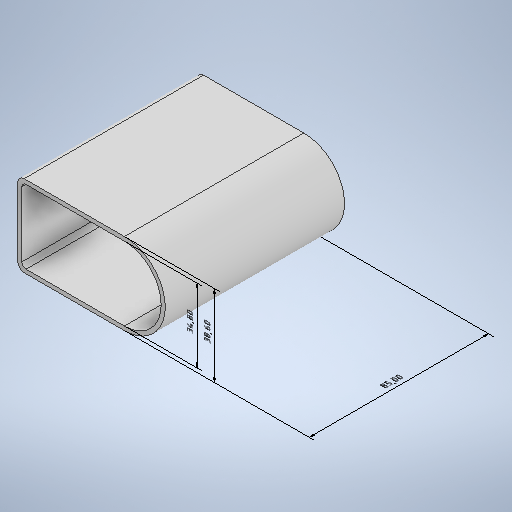
# Autodesk Inventor part: víko
Saved by Autodesk Inventor 2025.3 (Build 293356000, 356)
## iProperties
Created: 2025-06-12
Part Number: víko
Material: Generic
Document SubType Name: Modeling
Designer: Repete
Density: 1 g/cm^3
Appearance: Default
Author: Repete
Autodesk Inventor part; units mm, degrees
ref_plane "YZ Plane" through (0, 0, 0) normal (1, 0, 0) x (0, 1, 0)
ref_plane "XZ Plane" through (0, 0, 0) normal (0, 1, 0) x (-1, 0, 0)
ref_plane "XY Plane" through (0, 0, 0) normal (0, 0, 1) x (1, 0, 0)
sketch "Sketch1" plane through (0, 0, 0) normal (0, 1, 0) x (-1, 0, 0)
  line L0 (35.4, 17.4) -> (35.4, -17.4)
  line L1 (35.4, -17.4) -> (-13.2013, -17.4)
  arc A0 (-13.2013, 17.4) -> (-13.2013, -17.4) centre (-13.2013, 0) ccw
  line L2 (-13.2013, 17.4) -> (35.4, 17.4)
  line L3 (37.3, -19.3) -> (37.3, 19.3)
  line L4 (37.3, 19.3) -> (-13.2013, 19.3)
  arc A1 (-13.2013, 19.3) -> (-13.2013, -19.3) centre (-13.2013, 0) ccw
  line L5 (-13.2013, -19.3) -> (37.3, -19.3)
  point P0 (0, 0)
  point P1 (-13.2013, 0)
  point P2 (0, 0)
  point P3 (-12.8411, -36.7096)
  point P4 (-12.8411, -7.716)
  point P5 (-24.0253, -72.4098)
  constraints: 12 end point, 4 point on circle, 2 centre point, 2 parallel, 2 perpendicular
extrude "Extrusion1" add sketch "Sketch1" along normal blind 83
ref_plane "Work Plane1" through (0, 85, 0) normal (0, 1, 0) x (1, 0, 0)
sketch "Sketch2" plane through (0, 85, 0) normal (0, 1, 0) x (1, 0, 0)
  line L0 (-37.3, 19.3) -> (-37.3, -19.3)
  line L1 (-37.3, -19.3) -> (13.2013, -19.3)
  arc A0 (13.2013, -19.3) -> (13.2013, 19.3) centre (13.2013, 0) ccw
  line L2 (13.2013, 19.3) -> (-37.3, 19.3)
  point P0 (0, 0)
  point P1 (0, 0)
  point P2 (13.2013, 0)
  point P3 (0, 0)
  point P4 (14.0497, 95.3418)
  point P5 (14.0497, 124.3354)
  point P6 (2.8654, 59.6417)
  constraints: 6 end point, 2 point on circle, 1 centre point, 1 parallel, 1 perpendicular
extrude "Extrusion2" add sketch "Sketch2" against normal up to surface (2 mm away)
fillet "Fillet1" radius 3 3 edges at (-37.3, 41.5, -19.3) (-37.3, 84, -19.3) (-37.3, 42.5, 19.3)
fillet "Fillet2" radius 2 2 edges at (-35.4, 41.5, -17.4) (-35.4, 41.5, 17.4)
body "Solid1"
